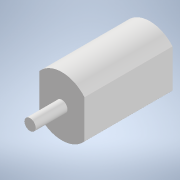
# Autodesk Inventor part: motor_12v
Saved by Autodesk Inventor 2022 (Build 260153000, 153)
## iProperties
Created: 2022-03-16
Part Number: motor_12v
Material: Generic
Document SubType Name: Modeling
Designer: katha
Density: 1 g/cm^3
Appearance: Default
Author: katha
Autodesk Inventor part; units mm, degrees
ref_plane "YZ Plane" through (0, 0, 0) normal (1, 0, 0) x (0, 1, 0)
ref_plane "XZ Plane" through (0, 0, 0) normal (0, 1, 0) x (-1, 0, 0)
ref_plane "XY Plane" through (0, 0, 0) normal (0, 0, 1) x (1, 0, 0)
sketch "Sketch1" plane through (0, 0, 0) normal (0, 0, 1) x (1, 0, 0)
  line L0 (91.3955, 137.1362) -> (100.6455, 137.1362) construction
  line L1 (100.6455, 137.1362) -> (100.6455, 129.3358)
  line L2 (100.6455, 137.1362) -> (100.6455, 144.9367)
  line L3 (91.3955, 137.1362) -> (91.3955, 122.6202) construction
  line L4 (82.1455, 137.1362) -> (82.1455, 129.3358)
  line L5 (82.1455, 137.1362) -> (82.1455, 144.9367)
  arc A0 (100.6455, 144.9367) -> (82.1455, 144.9367) centre (91.3955, 137.1362) ccw
  arc A1 (82.1455, 129.3358) -> (100.6455, 129.3358) centre (91.3955, 137.1362) ccw
  point P0 (0, 0)
  point P1 (100.6455, 120.0736)
  point P2 (100.6455, 151.3606)
  point P3 (82.1455, 120.0736)
  point P4 (82.1455, 151.3606)
  dimension "d1" = 9.25
  constraints: 12 end point, 4 point on circle, 3 symmetric about line, 3 vertical, 2 centre point, 1 horizontal
  measures "d1" distance of L0.start L0.end
extrude "Extrusion1" add sketch "Sketch1" along normal blind 36
sketch "Sketch2" plane through (0, 0, 36) normal (0, 0, 1) x (1, 0, 0)
  arc A0 (100.6455, 144.9367) -> (82.1455, 144.9367) centre (91.3955, 137.1362) ccw projected
  circle A1 centre (91.3955, 137.1362) radius 2.3
  point P0 (0, 0)
  dimension "d4" = 4.6
  constraints: 1 centre point, 1 coincident
  measures "d4" diameter of A1
extrude "Extrusion2" add sketch "Sketch2" along normal blind 13
body "Solid1"
